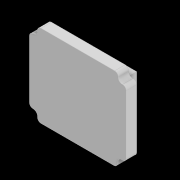
# Autodesk Inventor part: switchback-logo
Saved by Autodesk Inventor 2020 (Build 240168000, 168)
## iProperties
Created: 2020-02-04
Part Number: switchback-logo
Material: Generic
Document SubType Name: Modeling
Designer: valer
Density: 1 g/cm^3
Appearance: Default
Author: valer
Autodesk Inventor part; units mm, degrees
ref_plane "YZ Plane" through (0, 0, 0) normal (1, 0, 0) x (0, 1, 0)
ref_plane "XZ Plane" through (0, 0, 0) normal (0, 1, 0) x (-1, 0, 0)
ref_plane "XY Plane" through (0, 0, 0) normal (0, 0, 1) x (1, 0, 0)
sketch "Base" plane through (0, 0, 0) normal (0, 0, 1) x (1, 0, 0)
  spline S0 degree 3 poles (29.6992, 1.1773) (29.7109, 1.3423) (29.6903, 1.508) (29.5867, 1.8221) (29.5048, 1.9675) (29.2897, 2.2188) (29.1586, 2.3222) (28.9221, 2.4433) (28.8277, 2.4783) (28.6327, 2.5254) (28.5327, 2.5373) (28.4324, 2.5373) knots 0 0 0 0 0.049612 0.049612 0.099224 0.099224 0.148836 0.148836 0.178932 0.178932 0.209028 0.209028 0.209028 0.209028
  line L0 (1.5557, 2.5369) -> (28.4324, 2.5373)
  spline S1 degree 3 poles (1.5557, 2.5369) (1.3904, 2.5369) (1.2266, 2.5046) (0.9206, 2.379) (0.7813, 2.287) (0.5459, 2.0546) (0.452, 1.9166) (0.3443, 1.6634) (0.3145, 1.5572) (0.2831, 1.3399) (0.2816, 1.2297) (0.2942, 1.1206) knots 0 0 0 0 0.049612 0.049612 0.099224 0.099224 0.148836 0.148836 0.181775 0.181775 0.214715 0.214715 0.214715 0.214715
  arc A0 (0, 0) -> (0.2942, 1.1206) centre (-1.2879, 0.9371) ccw
  line L1 (30.1691, 0) -> (0, 0)
  arc A1 (29.6992, 1.1773) -> (30.1691, 0) centre (31.151, 1.0743) ccw
  spline S2 degree 3 poles (-2.6437, -23.0226) (-2.6437, -23.1879) (-2.6114, -23.3517) (-2.4858, -23.6576) (-2.3938, -23.7968) (-2.1615, -24.0323) (-2.0234, -24.1261) (-1.7866, -24.227) (-1.6982, -24.2538) (-1.5172, -24.2877) (-1.4252, -24.2948) (-1.3332, -24.2919) knots 0 0 0 0 0.049602 0.049602 0.099207 0.099207 0.148822 0.148822 0.176438 0.176438 0.204053 0.204053 0.204053 0.204053
  arc A2 (0, -24.9362) -> (-1.3332, -24.2919) centre (-1.2826, -25.8888) ccw
  line L2 (0, 0) -> (0, -24.9362)
  arc A3 (-1.3355, -0.6549) -> (0, 0) centre (-1.2879, 0.9371) ccw
  spline S3 degree 3 poles (-1.3355, -0.6549) (-1.5008, -0.65) (-1.6656, -0.6774) (-1.9753, -0.7938) (-2.1173, -0.8817) (-2.3596, -1.107) (-2.4576, -1.2422) (-2.5652, -1.4755) (-2.5945, -1.5626) (-2.6338, -1.7415) (-2.6437, -1.8328) (-2.6437, -1.9244) knots 0 0 0 0 0.049634 0.049634 0.099263 0.099263 0.148881 0.148881 0.176354 0.176354 0.203827 0.203827 0.203827 0.203827
  line L3 (-2.6437, -23.0226) -> (-2.6437, -1.9244)
  spline S4 degree 3 poles (28.1591, -27.4789) (28.3245, -27.4789) (28.4883, -27.4466) (28.7943, -27.3211) (28.9335, -27.229) (29.1689, -26.9966) (29.2628, -26.8586) (29.3703, -26.6061) (29.3999, -26.5007) (29.4315, -26.285) (29.4334, -26.1755) (29.4212, -26.0671) knots 0 0 0 0 0.049612 0.049612 0.099224 0.099224 0.148836 0.148836 0.181546 0.181546 0.214256 0.214256 0.214256 0.214256
  arc A4 (31.1912, -24.3016) -> (29.4212, -26.0671) centre (31.0088, -25.8888) ccw
  spline S5 degree 3 poles (31.1912, -24.3016) (31.3556, -24.3204) (31.5221, -24.307) (31.8405, -24.2172) (31.9894, -24.1416) (32.2499, -23.9376) (32.3589, -23.8111) (32.4948, -23.5721) (32.5363, -23.4703) (32.5923, -23.2585) (32.6065, -23.1495) (32.6065, -23.0399) knots 0 0 0 0 0.049634 0.049634 0.099263 0.099263 0.148881 0.148881 0.18174 0.18174 0.214599 0.214599 0.214599 0.214599
  line L4 (32.6065, -1.6448) -> (32.6065, -23.0399)
  spline S6 degree 3 poles (32.6065, -1.6448) (32.6065, -1.4795) (32.5742, -1.3157) (32.4486, -1.0098) (32.3566, -0.8705) (32.1243, -0.6351) (31.9862, -0.5412) (31.7423, -0.4373) (31.6462, -0.4092) (31.4495, -0.376) (31.3495, -0.371) (31.2499, -0.3778) knots 0 0 0 0 0.049602 0.049602 0.099206 0.099206 0.14882 0.14882 0.178752 0.178752 0.208681 0.208681 0.208681 0.208681
  arc A5 (30.1691, 0) -> (31.2499, -0.3778) centre (31.151, 1.0743) ccw
  line L5 (30.1691, -22.3113) -> (30.1691, 0)
  line L6 (27.5442, -22.3113) -> (30.1691, -22.3113)
  line L7 (27.5442, -24.9362) -> (27.5442, -22.3113)
  line L8 (0, -24.9362) -> (27.5442, -24.9362)
  arc A6 (0.305, -26.0673) -> (0, -24.9362) centre (-1.2826, -25.8888) ccw
  spline S7 degree 3 poles (0.305, -26.0673) (0.2866, -26.2317) (0.3003, -26.398) (0.3909, -26.7161) (0.4669, -26.8648) (0.6714, -27.1247) (0.7981, -27.2334) (1.037, -27.3685) (1.1385, -27.4097) (1.3494, -27.4652) (1.458, -27.4793) (1.5671, -27.4793) knots 0 0 0 0 0.049612 0.049612 0.099224 0.099224 0.148836 0.148836 0.181555 0.181555 0.214273 0.214273 0.214273 0.214273
  line L9 (28.1591, -27.4789) -> (1.5671, -27.4793)
  point P0 (30.1691, 0)
  point P1 (30.1691, 0)
  constraints: 20 end point, 14 point on circle, 7 centre point, 16 other
extrude "BaseFeature" add sketch "Base" along normal blind 3.81
extrude "LogoFeature" add sketch "Base" against normal blind 5.08 contours L5 L6 L7 L8 L2 L1
sketch "LogoDetail" plane through (0, 0, -5.08) normal (0, 0, -1) x (-1, 0, 0)
  line L0 (-18.374, -7.8746) -> (-22.2945, -7.8746)
  line L1 (-27.5442, -22.3113) -> (-13.1243, -22.3113)
  line L2 (-22.2945, -17.0616) -> (-18.374, -17.0616)
  line L3 (-13.1243, -2.6249) -> (-27.5442, -2.6249)
  line L4 (-22.2945, -7.8746) -> (-22.2945, -17.0616)
  line L5 (-18.374, -17.0616) -> (-18.374, -7.8746)
  line L6 (-30.1691, -22.3113) -> (-30.1691, 0)
  line L7 (-27.5442, -2.6249) -> (-27.5442, -22.3113)
  line L8 (-13.1243, -22.3113) -> (-13.1243, -2.6249)
  line L9 (-30.1691, 0) -> (0, 0)
  line L10 (0, -24.9362) -> (-27.5442, -24.9362)
  line L11 (-7.8746, -2.6249) -> (-7.8746, -22.3113)
  line L12 (-2.6249, -22.3113) -> (-2.6249, -2.6249)
  line L13 (-7.8746, -22.3113) -> (-2.6249, -22.3113)
  line L14 (-2.6249, -2.6249) -> (-7.8746, -2.6249)
  line L15 (-27.5442, -24.9362) -> (-27.5442, -22.3113)
  line L16 (-27.5442, -22.3113) -> (-30.1691, -22.3113)
  line L17 (0, 0) -> (0, -24.9362)
  line L18 (-30.1691, -22.3113) -> (-30.1691, -24.9362)
  line L19 (-30.1691, -24.9362) -> (-27.5442, -24.9362)
  line L20 (0, 0) -> (-30.1691, 0) projected
  line L21 (-30.1691, 0) -> (-30.1691, -22.3113) projected
  dimension "d4" = 3.9205
  dimension "d5" = 5.2497
  dimension "d6" = 5.2497
  dimension "d7" = 5.2497
  dimension "d8" = 2.6249
  dimension "d9" = 5.2497
  dimension "d10" = 5.2497
  dimension "d11" = 2.6249
  dimension "d12" = 2.6249
  dimension "d13" = 2.6249
  dimension "d14" = 24.9362
  dimension "d15" = 27.5443
  dimension "d16" = 5.2497
  constraints: 40 end point, 7 perpendicular, 5 collinear, 3 parallel, 1 coincident, 1 horizontal, 1 vertical
  measures "d4" distance between parallel lines of L4 L5
  measures "d5" distance between parallel lines of L4 L7
  measures "d6" distance between parallel lines of L12 L11
  measures "d7" distance between parallel lines of L11 L8
  measures "d8" distance between parallel lines of L9 L3
  measures "d9" distance between parallel lines of L8 L5
  measures "d10" distance between parallel lines of L1 L2
  measures "d11" distance between parallel lines of L10 L13
  measures "d12" distance between parallel lines of L17 L12
  measures "d13" distance between parallel lines of L6 L7
  measures "d14" distance of L9.end L17.end
  measures "d15" distance of L17.end L10.end
  measures "d16" distance between parallel lines of L3 L0
extrude "LogoDetailFeature" cut sketch "LogoDetail" against normal blind 5.08 contours L5 L2 L4 L0 | L16 L6 L9 L17 L10 L15
body "Solid1"
